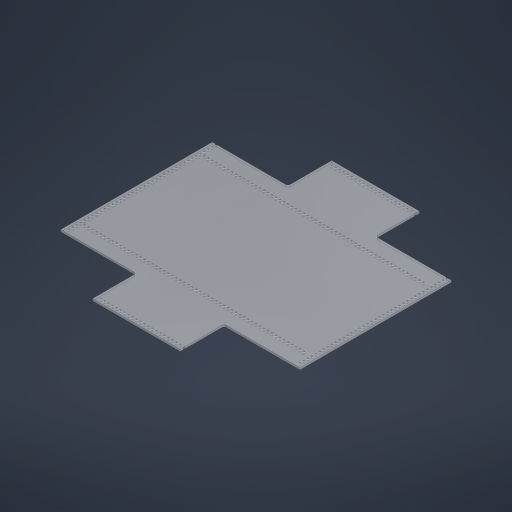
# Autodesk Inventor part: Belly Pan
Saved by Autodesk Inventor 2024.3 (Build 283343000, 343)
## iProperties
Created: 2024-11-27
Part Number: Belly Pan
Material: Generic
Document SubType Name: Modeling
Designer: kaito
Density: 1 g/cm^3
Appearance: Polycarbonate - Clear
Author: kaito
Autodesk Inventor part; units mm, degrees
ref_plane "YZ Plane" through (0, 0, 0) normal (1, 0, 0) x (0, 1, 0)
ref_plane "XZ Plane" through (0, 0, 0) normal (0, 1, 0) x (-1, 0, 0)
ref_plane "XY Plane" through (0, 0, 0) normal (0, 0, 1) x (1, 0, 0)
sketch "Sketch1" plane through (0, 0, 0) normal (0, 1, 0) x (-1, 0, 0)
  line L0 (0, 0) -> (762, 0) construction
  line L1 (762, 0) -> (762, -762)
  line L2 (762, -762) -> (0, -762)
  line L3 (762, -139.7) -> (736.6, -139.7) construction
  line L4 (736.6, -139.7) -> (736.6, -622.3) construction
  line L5 (736.6, -622.3) -> (762, -622.3) construction
  line L6 (762, -622.3) -> (762, -139.7) construction
  line L7 (520.7, 0) -> (241.3, 0)
  line L8 (241.3, 0) -> (241.3, -25.4) construction
  line L9 (241.3, -25.4) -> (520.7, -25.4) construction
  line L10 (520.7, -25.4) -> (520.7, 0) construction
  line L11 (520.7, -762) -> (241.3, -762) construction
  line L12 (241.3, -762) -> (241.3, -736.6) construction
  line L13 (241.3, -736.6) -> (520.7, -736.6) construction
  line L14 (520.7, -736.6) -> (520.7, -762) construction
  line L15 (0, 0) -> (0, -762)
  line L16 (0, -139.7) -> (25.4, -139.7) construction
  line L17 (25.4, -139.7) -> (25.4, -622.3) construction
  line L18 (25.4, -622.3) -> (0, -622.3) construction
  line L19 (0, -622.3) -> (0, -139.7) construction
  circle A0 centre (508, -12.7) radius 2.4892
  circle A1 centre (495.3, -12.7) radius 2.4892
  circle A2 centre (482.6, -12.7) radius 2.4892
  circle A3 centre (469.9, -12.7) radius 2.4892
  circle A4 centre (457.2, -12.7) radius 2.4892
  circle A5 centre (444.5, -12.7) radius 2.4892
  circle A6 centre (431.8, -12.7) radius 2.4892
  circle A7 centre (419.1, -12.7) radius 2.4892
  circle A8 centre (406.4, -12.7) radius 2.4892
  circle A9 centre (393.7, -12.7) radius 2.4892
  circle A10 centre (381, -12.7) radius 2.4892
  circle A11 centre (368.3, -12.7) radius 2.4892
  circle A12 centre (749.3, -152.4) radius 2.4892
  circle A13 centre (749.3, -165.1) radius 2.4892
  circle A14 centre (749.3, -177.8) radius 2.4892
  circle A15 centre (749.3, -190.5) radius 2.4892
  circle A16 centre (749.3, -203.2) radius 2.4892
  circle A17 centre (749.3, -215.9) radius 2.4892
  circle A18 centre (749.3, -228.6) radius 2.4892
  circle A19 centre (749.3, -241.3) radius 2.4892
  circle A20 centre (749.3, -254) radius 2.4892
  circle A21 centre (749.3, -266.7) radius 2.4892
  circle A22 centre (749.3, -279.4) radius 2.4892
  circle A23 centre (749.3, -292.1) radius 2.4892
  circle A24 centre (749.3, -304.8) radius 2.4892
  circle A25 centre (749.3, -317.5) radius 2.4892
  circle A26 centre (749.3, -330.2) radius 2.4892
  circle A27 centre (749.3, -342.9) radius 2.4892
  circle A28 centre (749.3, -355.6) radius 2.4892
  circle A29 centre (508, -749.3) radius 2.4892
  circle A30 centre (495.3, -749.3) radius 2.4892
  circle A31 centre (482.6, -749.3) radius 2.4892
  circle A32 centre (469.9, -749.3) radius 2.4892
  circle A33 centre (457.2, -749.3) radius 2.4892
  circle A34 centre (444.5, -749.3) radius 2.4892
  circle A35 centre (431.8, -749.3) radius 2.4892
  circle A36 centre (419.1, -749.3) radius 2.4892
  circle A37 centre (406.4, -749.3) radius 2.4892
  circle A38 centre (393.7, -749.3) radius 2.4892
  circle A39 centre (381, -749.3) radius 2.4892
  circle A40 centre (368.3, -749.3) radius 2.4892
  circle A41 centre (355.6, -749.3) radius 2.4892
  circle A42 centre (342.9, -749.3) radius 2.4892
  circle A43 centre (330.2, -749.3) radius 2.4892
  circle A44 centre (317.5, -749.3) radius 2.4892
  circle A45 centre (304.8, -749.3) radius 2.4892
  line L20 (762, 0) -> (520.7, 0)
  line L21 (520.7, 0) -> (520.7, -132.08)
  line L22 (528.32, -139.7) -> (762, -139.7)
  line L23 (762, -139.7) -> (762, 0)
  line L24 (762, -622.3) -> (528.32, -622.3)
  line L25 (520.7, -629.92) -> (520.7, -762)
  line L26 (520.7, -762) -> (762, -762)
  line L27 (762, -762) -> (762, -622.3)
  line L28 (241.3, -762) -> (0, -762)
  line L29 (0, -762) -> (0, -622.3)
  line L30 (0, -622.3) -> (233.68, -622.3)
  line L31 (241.3, -629.92) -> (241.3, -762)
  line L32 (241.3, 0) -> (0, 0)
  line L33 (0, 0) -> (0, -139.7)
  line L34 (0, -139.7) -> (233.68, -139.7)
  line L35 (241.3, -132.08) -> (241.3, 0)
  circle A46 centre (749.3, -368.3) radius 2.4892
  circle A47 centre (749.3, -381) radius 2.4892
  circle A48 centre (749.3, -393.7) radius 2.4892
  circle A49 centre (749.3, -406.4) radius 2.4892
  circle A50 centre (749.3, -419.1) radius 2.4892
  circle A51 centre (749.3, -431.8) radius 2.4892
  circle A52 centre (749.3, -444.5) radius 2.4892
  circle A53 centre (749.3, -457.2) radius 2.4892
  circle A54 centre (749.3, -469.9) radius 2.4892
  circle A55 centre (749.3, -482.6) radius 2.4892
  circle A56 centre (749.3, -495.3) radius 2.4892
  circle A57 centre (749.3, -508) radius 2.4892
  circle A58 centre (749.3, -520.7) radius 2.4892
  circle A59 centre (749.3, -533.4) radius 2.4892
  circle A60 centre (749.3, -546.1) radius 2.4892
  circle A61 centre (749.3, -558.8) radius 2.4892
  circle A62 centre (749.3, -571.5) radius 2.4892
  circle A63 centre (749.3, -584.2) radius 2.4892
  circle A64 centre (749.3, -596.9) radius 2.4892
  circle A65 centre (749.3, -609.6) radius 2.4892
  circle A66 centre (749.3, -622.3) radius 2.4892
  circle A67 centre (12.7, -152.4) radius 2.4892
  circle A68 centre (12.7, -165.1) radius 2.4892
  circle A69 centre (12.7, -177.8) radius 2.4892
  circle A70 centre (12.7, -190.5) radius 2.4892
  circle A71 centre (12.7, -203.2) radius 2.4892
  circle A72 centre (12.7, -215.9) radius 2.4892
  circle A73 centre (12.7, -228.6) radius 2.4892
  circle A74 centre (12.7, -241.3) radius 2.4892
  circle A75 centre (12.7, -254) radius 2.4892
  circle A76 centre (12.7, -266.7) radius 2.4892
  circle A77 centre (12.7, -279.4) radius 2.4892
  circle A78 centre (12.7, -292.1) radius 2.4892
  circle A79 centre (12.7, -304.8) radius 2.4892
  circle A80 centre (12.7, -317.5) radius 2.4892
  circle A81 centre (12.7, -330.2) radius 2.4892
  circle A82 centre (12.7, -342.9) radius 2.4892
  circle A83 centre (12.7, -355.6) radius 2.4892
  circle A84 centre (12.7, -368.3) radius 2.4892
  circle A85 centre (12.7, -381) radius 2.4892
  circle A86 centre (12.7, -393.7) radius 2.4892
  circle A87 centre (12.7, -406.4) radius 2.4892
  circle A88 centre (12.7, -419.1) radius 2.4892
  circle A89 centre (12.7, -431.8) radius 2.4892
  circle A90 centre (12.7, -444.5) radius 2.4892
  circle A91 centre (12.7, -457.2) radius 2.4892
  circle A92 centre (12.7, -469.9) radius 2.4892
  circle A93 centre (12.7, -482.6) radius 2.4892
  circle A94 centre (12.7, -495.3) radius 2.4892
  circle A95 centre (12.7, -508) radius 2.4892
  circle A96 centre (12.7, -520.7) radius 2.4892
  circle A97 centre (12.7, -533.4) radius 2.4892
  circle A98 centre (12.7, -546.1) radius 2.4892
  circle A99 centre (12.7, -558.8) radius 2.4892
  circle A100 centre (12.7, -571.5) radius 2.4892
  circle A101 centre (12.7, -584.2) radius 2.4892
  circle A102 centre (12.7, -596.9) radius 2.4892
  circle A103 centre (12.7, -609.6) radius 2.4892
  circle A104 centre (12.7, -622.3) radius 2.4892
  circle A105 centre (355.6, -12.7) radius 2.4892
  circle A106 centre (342.9, -12.7) radius 2.4892
  circle A107 centre (330.2, -12.7) radius 2.4892
  circle A108 centre (317.5, -12.7) radius 2.4892
  circle A109 centre (304.8, -12.7) radius 2.4892
  circle A110 centre (292.1, -12.7) radius 2.4892
  circle A111 centre (279.4, -12.7) radius 2.4892
  circle A112 centre (266.7, -12.7) radius 2.4892
  circle A113 centre (254, -12.7) radius 2.4892
  circle A114 centre (241.3, -12.7) radius 2.4892
  circle A115 centre (292.1, -749.3) radius 2.4892
  circle A116 centre (279.4, -749.3) radius 2.4892
  circle A117 centre (266.7, -749.3) radius 2.4892
  circle A118 centre (254, -749.3) radius 2.4892
  circle A119 centre (241.3, -749.3) radius 2.4892
  arc A120 (528.32, -622.3) -> (520.7, -629.92) centre (528.32, -629.92) ccw
  arc A121 (241.3, -629.92) -> (233.68, -622.3) centre (233.68, -629.92) ccw
  arc A122 (520.7, -132.08) -> (528.32, -139.7) centre (528.32, -132.08) ccw
  arc A123 (233.68, -139.7) -> (241.3, -132.08) centre (233.68, -132.08) ccw
  line L36 (25.4, -177.8029) -> (736.6, -177.8029) construction
  line L37 (736.6, -177.8029) -> (736.6, -203.2029) construction
  line L38 (736.6, -203.2029) -> (25.4, -203.2029) construction
  line L39 (25.4, -203.2029) -> (25.4, -177.8029) construction
  circle A124 centre (38.1, -190.5029) radius 2.4892
  circle A125 centre (50.8, -190.5029) radius 2.4892
  circle A126 centre (63.5, -190.5029) radius 2.4892
  circle A127 centre (76.2, -190.5029) radius 2.4892
  circle A128 centre (88.9, -190.5029) radius 2.4892
  circle A129 centre (101.6, -190.5029) radius 2.4892
  circle A130 centre (114.3, -190.5029) radius 2.4892
  circle A131 centre (127, -190.5029) radius 2.4892
  circle A132 centre (139.7, -190.5029) radius 2.4892
  circle A133 centre (152.4, -190.5029) radius 2.4892
  circle A134 centre (165.1, -190.5029) radius 2.4892
  circle A135 centre (177.8, -190.5029) radius 2.4892
  circle A136 centre (190.5, -190.5029) radius 2.4892
  circle A137 centre (203.2, -190.5029) radius 2.4892
  circle A138 centre (215.9, -190.5029) radius 2.4892
  circle A139 centre (228.6, -190.5029) radius 2.4892
  circle A140 centre (241.3, -190.5029) radius 2.4892
  circle A141 centre (254, -190.5029) radius 2.4892
  circle A142 centre (266.7, -190.5029) radius 2.4892
  circle A143 centre (279.4, -190.5029) radius 2.4892
  circle A144 centre (292.1, -190.5029) radius 2.4892
  circle A145 centre (304.8, -190.5029) radius 2.4892
  circle A146 centre (317.5, -190.5029) radius 2.4892
  circle A147 centre (330.2, -190.5029) radius 2.4892
  circle A148 centre (342.9, -190.5029) radius 2.4892
  circle A149 centre (355.6, -190.5029) radius 2.4892
  circle A150 centre (368.3, -190.5029) radius 2.4892
  circle A151 centre (381, -190.5029) radius 2.4892
  circle A152 centre (393.7, -190.5029) radius 2.4892
  circle A153 centre (406.4, -190.5029) radius 2.4892
  circle A154 centre (419.1, -190.5029) radius 2.4892
  circle A155 centre (431.8, -190.5029) radius 2.4892
  circle A156 centre (444.5, -190.5029) radius 2.4892
  circle A157 centre (457.2, -190.5029) radius 2.4892
  circle A158 centre (469.9, -190.5029) radius 2.4892
  circle A159 centre (482.6, -190.5029) radius 2.4892
  circle A160 centre (495.3, -190.5029) radius 2.4892
  circle A161 centre (508, -190.5029) radius 2.4892
  circle A162 centre (520.7, -190.5029) radius 2.4892
  circle A163 centre (533.4, -190.5029) radius 2.4892
  circle A164 centre (546.1, -190.5029) radius 2.4892
  circle A165 centre (558.8, -190.5029) radius 2.4892
  circle A166 centre (571.5, -190.5029) radius 2.4892
  circle A167 centre (584.2, -190.5029) radius 2.4892
  circle A168 centre (596.9, -190.5029) radius 2.4892
  circle A169 centre (609.6, -190.5029) radius 2.4892
  circle A170 centre (622.3, -190.5029) radius 2.4892
  circle A171 centre (635, -190.5029) radius 2.4892
  circle A172 centre (647.7, -190.5029) radius 2.4892
  circle A173 centre (660.4, -190.5029) radius 2.4892
  circle A174 centre (673.1, -190.5029) radius 2.4892
  circle A175 centre (685.8, -190.5029) radius 2.4892
  circle A176 centre (698.5, -190.5029) radius 2.4892
  circle A177 centre (711.2, -190.5029) radius 2.4892
  circle A178 centre (723.9, -190.5029) radius 2.4892
  circle A179 centre (736.6, -190.5029) radius 2.4892
  line L40 (25.4, -558.8) -> (736.6, -558.8) construction
  line L41 (736.6, -558.8) -> (736.6, -584.2) construction
  line L42 (736.6, -584.2) -> (25.4, -584.2) construction
  line L43 (25.4, -584.2) -> (25.4, -558.8) construction
  circle A180 centre (38.1, -571.5) radius 2.4892
  circle A181 centre (50.8, -571.5) radius 2.4892
  circle A182 centre (63.5, -571.5) radius 2.4892
  circle A183 centre (76.2, -571.5) radius 2.4892
  circle A184 centre (88.9, -571.5) radius 2.4892
  circle A185 centre (101.6, -571.5) radius 2.4892
  circle A186 centre (114.3, -571.5) radius 2.4892
  circle A187 centre (127, -571.5) radius 2.4892
  circle A188 centre (139.7, -571.5) radius 2.4892
  circle A189 centre (152.4, -571.5) radius 2.4892
  circle A190 centre (165.1, -571.5) radius 2.4892
  circle A191 centre (177.8, -571.5) radius 2.4892
  circle A192 centre (190.5, -571.5) radius 2.4892
  circle A193 centre (203.2, -571.5) radius 2.4892
  circle A194 centre (215.9, -571.5) radius 2.4892
  circle A195 centre (228.6, -571.5) radius 2.4892
  circle A196 centre (241.3, -571.5) radius 2.4892
  circle A197 centre (254, -571.5) radius 2.4892
  circle A198 centre (266.7, -571.5) radius 2.4892
  circle A199 centre (279.4, -571.5) radius 2.4892
  circle A200 centre (292.1, -571.5) radius 2.4892
  circle A201 centre (304.8, -571.5) radius 2.4892
  circle A202 centre (317.5, -571.5) radius 2.4892
  circle A203 centre (330.2, -571.5) radius 2.4892
  circle A204 centre (342.9, -571.5) radius 2.4892
  circle A205 centre (355.6, -571.5) radius 2.4892
  circle A206 centre (368.3, -571.5) radius 2.4892
  circle A207 centre (381, -571.5) radius 2.4892
  circle A208 centre (393.7, -571.5) radius 2.4892
  circle A209 centre (406.4, -571.5) radius 2.4892
  circle A210 centre (419.1, -571.5) radius 2.4892
  circle A211 centre (431.8, -571.5) radius 2.4892
  circle A212 centre (444.5, -571.5) radius 2.4892
  circle A213 centre (457.2, -571.5) radius 2.4892
  circle A214 centre (469.9, -571.5) radius 2.4892
  circle A215 centre (482.6, -571.5) radius 2.4892
  circle A216 centre (495.3, -571.5) radius 2.4892
  circle A217 centre (508, -571.5) radius 2.4892
  circle A218 centre (520.7, -571.5) radius 2.4892
  circle A219 centre (533.4, -571.5) radius 2.4892
  circle A220 centre (546.1, -571.5) radius 2.4892
  circle A221 centre (558.8, -571.5) radius 2.4892
  circle A222 centre (571.5, -571.5) radius 2.4892
  circle A223 centre (584.2, -571.5) radius 2.4892
  circle A224 centre (596.9, -571.5) radius 2.4892
  circle A225 centre (609.6, -571.5) radius 2.4892
  circle A226 centre (622.3, -571.5) radius 2.4892
  circle A227 centre (635, -571.5) radius 2.4892
  circle A228 centre (647.7, -571.5) radius 2.4892
  circle A229 centre (660.4, -571.5) radius 2.4892
  circle A230 centre (673.1, -571.5) radius 2.4892
  circle A231 centre (685.8, -571.5) radius 2.4892
  circle A232 centre (698.5, -571.5) radius 2.4892
  circle A233 centre (711.2, -571.5) radius 2.4892
  circle A234 centre (723.9, -571.5) radius 2.4892
  circle A235 centre (736.6, -571.5) radius 2.4892
  point P0 (736.6, -381)
  point P1 (381, -25.4)
  point P2 (381, 0)
  point P3 (381, -736.6)
  point P4 (381, -762)
  point P5 (25.4, -381)
  point P6 (0, -381)
  point P7 (762, -381)
  point P8 (12.7, -139.7)
  point P9 (12.7, -622.3)
  point P10 (520.7, -12.7)
  point P11 (749.3, -139.7)
  point P12 (520.7, -749.3)
  point P13 (0, -381)
  point P14 (520.7, -139.7)
  point P15 (25.4, -190.5029)
  point P16 (25.4, -571.5)
  dimension "d0" = 762
  dimension "d1" = 762
  dimension "d4" = 25.4
  dimension "d6" = 25.4
  dimension "d7" = 279.4
  dimension "d8" = 25.4
  dimension "d9" = 25.4
  dimension "d11" = 482.6
  dimension "d22" = 4.9784
  dimension "d26" = 12.7
  dimension "d31" = 4.9784
  dimension "d32" = 12.7
  dimension "d35" = 12.7
  dimension "d40" = 4.9784
  dimension "d41" = 12.7
  dimension "d44" = 12.7
  dimension "d51" = 482.6
  dimension "d382" = 139.7
  dimension "d383" = 279.4
  dimension "d384" = 4.9784
  dimension "d387" = 12.7
  dimension "d392" = 7.62
  dimension "d393" = 7.62
  dimension "d396" = 177.8029
  dimension "d397" = 25.4
  dimension "d398" = 4.9784
  dimension "d399" = 12.7
  dimension "d402" = 12.7
  dimension "d407" = 25.4
  dimension "d408" = 177.8
  dimension "d409" = 4.9784
  dimension "d410" = 12.7
  dimension "d413" = 12.7
  dimension "d418" = 279.4
  dimension "d419" = 12.7
  constraints: 236 centre point, 88 end point, 21 parallel, 16 midpoint, 15 horizontal, 11 perpendicular, 10 point on line, 8 point on circle, 8 tangent, 7 horizontal alignment, 4 vertical alignment, 3 vertical, 2 equal radius, 452 other
  measures "d0" distance of L1.end L2.end
  measures "d1" distance of L0.end L1.end
  measures "d4" distance of L5.end L4.end
  measures "d6" distance of L8.end L7.end
  measures "d7" distance of L12.end L13.end
  measures "d8" distance of L11.end L12.end
  measures "d9" distance of L17.end L18.end
  measures "d11" distance of L3.end L4.end
  measures "d22" diameter of A0
  measures "d26" distance of A0.centre A1.centre
  measures "d31" diameter of A12
  measures "d32" distance of point (749.3, -139.7) A12.centre
  measures "d35" distance of A12.centre A13.centre
  measures "d40" diameter of A29
  measures "d41" distance of A29.centre point (520.7, -749.3)
  measures "d44" distance of A29.centre A30.centre
  measures "d51" distance of L16.end L17.end
  measures "d382" distance of L20.end point (520.7, -139.7)
  measures "d383" distance between parallel lines of L35 L21
  measures "d384" diameter of A67
  measures "d387" distance of A67.centre A68.centre
  measures "d392" radius of A120
  measures "d393" radius of A121
  measures "d396" distance between parallel lines of L0 L36
  measures "d397" distance of L36.end L37.end
  measures "d398" diameter of A124
  measures "d399" distance of point (25.4, -190.503) A124.centre
  measures "d402" distance of A124.centre A125.centre
  measures "d407" distance of L40.end L41.end
  measures "d408" distance between parallel lines of L2 L42
  measures "d409" diameter of A180
  measures "d410" distance of point (25.4, -571.5) A180.centre
  measures "d413" distance of A180.centre A181.centre
  measures "d418" distance of L8.end L9.end
  measures "d419" distance of point (520.7, -12.7) A0.centre
extrude "Extrusion2" add sketch "Sketch1" along normal blind 6.35 contours L1 L24 A66 A120 L25 L2 L31 A119 A121 L30 A104 L15 L34 A123 L35 A114 L7 L21 A122 L22
body "Solid2"
